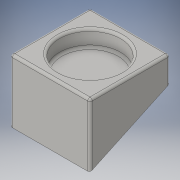
# Autodesk Inventor part: ChickenCupHolder
Saved by Autodesk Inventor 2016 (Build 200138000, 138)
## iProperties
Created: 2015-08-27
Part Number: ChickenCupHolder
Material: Generic
Document SubType Name: Modeling
Designer: steele
Density: 1 g/cm^3
Appearance: Default
Author: steele
Autodesk Inventor part; units mm, degrees
ref_plane "YZ Plane" through (0, 0, 0) normal (1, 0, 0) x (0, 1, 0)
ref_plane "XZ Plane" through (0, 0, 0) normal (0, 1, 0) x (-1, 0, 0)
ref_plane "XY Plane" through (0, 0, 0) normal (0, 0, 1) x (1, 0, 0)
sketch "Sketch1" plane through (0, 0, 0) normal (1, 0, 0) x (0, 1, 0)
  line L0 (0, 0) -> (-50.3379, 107.95)
  line L1 (-50.3379, 107.95) -> (34.925, 107.95)
  line L2 (34.925, 107.95) -> (34.925, 0)
  line L3 (34.925, 0) -> (0, 0)
  line L4 (0, 0) -> (0, 107.95) construction
  dimension "tilt" = 25
  dimension "baseDepth" = 107.95
  dimension "holderHeight" = 34.925
  constraints: 10 end point, 3 perpendicular, 1 horizontal, 1 point on line
  measures "tilt" angle of L4 L0
  measures "baseDepth" distance of L1.end L2.end
  measures "holderHeight" distance of L2.end L0.start
extrude "Extrusion1" add sketch "Sketch1" along normal mid plane 107.95
sketch "Sketch2" plane through (-53.975, 34.925, 107.95) normal (0, 1, 0) x (1, 0, 0)
  line L0 (107.95, 0) -> (0, 0) construction
  line L1 (107.95, 0) -> (107.95, 107.95) construction
  line L2 (0, 0) -> (107.95, 107.95) construction
  line L3 (0, 107.95) -> (107.95, 107.95) construction
  line L4 (0, 107.95) -> (107.95, 0) construction
  circle A0 centre (53.975, 53.975) radius 41.275
  point P0 (53.975, 107.95)
  dimension "d5" = 82.55
  constraints: 4 end point, 1 centre point, 1 midpoint
  measures "d5" diameter of A0
extrude "Extrusion2" cut sketch "Sketch2" against normal blind 22.225
sketch "Sketch4" plane through (-53.975, 0, 0) normal (0, -0.9063078, -0.4226183) x (1, 0, 0)
  line L0 (107.95, 119.1096) -> (107.95, 0) construction
  line L1 (107.95, 119.1096) -> (0, 119.1096) construction
  line L2 (107.95, 0) -> (0, 119.1096) construction
  line L3 (0, 0) -> (107.95, 0) construction
  line L4 (0, 0) -> (107.95, 119.1096) construction
  circle A0 centre (53.975, 59.5548) radius 41.275 construction
  ellipse E0 centre (53.975, 43.5507) end of major axis (12.7, 43.5507) minor radius 37.4079 projected
  point P0 (53.975, 0)
  point P1 (81.6929, 90.1382)
  point P2 (81.6929, 28.9715)
  point P3 (26.2571, 28.9715)
  point P4 (26.2571, 90.1382)
  dimension "d14" = 82.55
  constraints: 4 end point, 4 point on circle, 4 point on line, 1 centre point, 1 midpoint, 1 other
  measures "d14" diameter of A0
hole "Hole2" at (27.7179, -38.094, 81.6929) at (27.7179, -12.2439, 26.2571) at (-27.7179, -12.2439, 26.2571) at (-27.7179, -38.094, 81.6929) direction (0, 0.9063078, 0.4226183) diameter 7.7978 depth 22.225 tip angle 118 thread size "3/8-16 UNC" class "2B" standard "ANSI Unified Screw Threads"
fillet "Fillet1" radius 3.175 2 edges at (-41.275, 34.925, 53.975) (-41.275, 12.7, 53.975)
fillet "Fillet2" radius 3.175 4 edges at (0, 34.925, 107.95) (-53.975, 34.925, 53.975) (0, 34.925, 0) (53.975, 34.925, 53.975)
fillet "Fillet3" radius 3.175 8 edges at (-53.0451, 33.9951, 107.0201) (-53.975, -9.294, 107.95) (53.0451, 33.9951, 107.0201) (53.975, -9.294, 107.95) (53.0451, 33.9951, 0.9299) (53.975, 15.875, 0) (-53.0451, 33.9951, 0.9299) (-53.975, 15.875, 0)
equation "\"d5\" = cupDiam"
equation "\"d6\" = cupDepth"
equation "\"d14\" = cupDiam"
equation "\"d27\" = threadHoleDepth"
equation "\"d29\" = filet"
equation "\"d30\" = filet"
equation "\"d31\" = filet"
equation "\"cupDiam\" = 82.55"
equation "\"cupDepth\" = 22.225"
equation "\"threadHoleDepth\" = 22.225"
equation "\"filet\" = 3.175"
body "Solid1"
